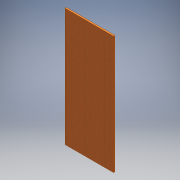
# Autodesk Inventor part: tapa
Saved by Autodesk Inventor 2016 (Build 200138000, 138)
## iProperties
Created: 2018-06-24
Part Number: tapa
Material: Wood (Cherry)
Document SubType Name: Modeling
Designer: damia
Density: 0.63 g/cm^3
Appearance: Cherry - Natural Low Gloss
Author: damia
Autodesk Inventor part; units mm, degrees
ref_plane "YZ Plane" through (0, 0, 0) normal (1, 0, 0) x (0, 1, 0)
ref_plane "XZ Plane" through (0, 0, 0) normal (0, 1, 0) x (-1, 0, 0)
ref_plane "XY Plane" through (0, 0, 0) normal (0, 0, 1) x (1, 0, 0)
sketch "Sketch1" plane through (0, 0, 0) normal (0, 1, 0) x (-1, 0, 0)
  line L0 (0, 0) -> (651, 0)
  line L1 (651, 0) -> (651, -1582)
  line L2 (651, -1582) -> (0, -1582)
  line L3 (0, -1582) -> (0, 0)
  dimension "d0" = 651
  dimension "d1" = 1582
  constraints: 8 end point, 2 parallel, 1 horizontal, 1 perpendicular
  measures "d0" distance of L1.end L2.end
  measures "d1" distance of L0.end L1.end
extrude "Extrusion1" add sketch "Sketch1" along normal blind 18
body "Solid1"
